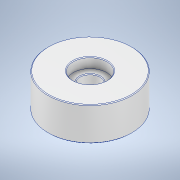
# Autodesk Inventor part: gegenroller
Saved by Autodesk Inventor 2022 (Build 260153000, 153)
## iProperties
Created: 2022-11-23
Part Number: gegenroller
Material: Aluminium 6061
Document SubType Name: Modeling
Designer: Friedrich Walmrath
Density: 2.7 g/cm^3
Appearance: Aluminium - flach
Author: Friedrich Walmrath
Autodesk Inventor part; units mm, degrees
ref_plane "YZ Plane" through (0, 0, 0) normal (1, 0, 0) x (0, 1, 0)
ref_plane "XZ Plane" through (0, 0, 0) normal (0, 1, 0) x (-1, 0, 0)
ref_plane "XY Plane" through (0, 0, 0) normal (0, 0, 1) x (1, 0, 0)
sketch "Skizze3" plane through (0, 0, 0) normal (0, 0, 1) x (1, 0, 0)
  line L0 (3, 3) -> (3, 7)
  line L1 (3, 7) -> (5, 7)
  line L2 (5, 7) -> (5, 10)
  line L3 (5, 10) -> (12.5, 10)
  line L4 (12.5, 10) -> (12.5, 0)
  line L5 (12.5, 0) -> (5, 0)
  line L6 (5, 0) -> (5, 3)
  line L7 (5, 3) -> (3, 3)
  line L8 (0, -2.8375) -> (0, 7.1625)
  point P0 (0, 0)
  dimension "d0" = 10
  dimension "d1" = 6
  dimension "d2" = 10
  dimension "d3" = 3
  dimension "d4" = 3
  dimension "d5" = 25
  constraints: 18 end point, 6 perpendicular, 3 point on line, 2 vertical, 1 horizontal alignment
  measures "d0" distance of L3.end L4.end
  measures "d1" diameter of L0 L8
  measures "d2" diameter of L2 L8
  measures "d3" distance of L1.end L2.end
  measures "d4" distance of L5.end L6.end
  measures "d5" diameter of L4 L8
revolve "Umdrehung1" add sketch "Skizze3" angle 360 about axis through (0, -2.8375, 0) along (0, 1, 0)
chamfer "Fase1" distance 0.2 angle 45 6 edges at (-12.5, 10, 0) (-12.5, 0, 0) (-3, 7, 0) (-5, 10, 0) (-3, 3, 0) (-5, 0, 0)
